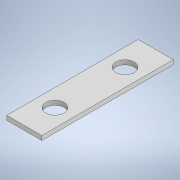
# Autodesk Inventor part: DrillSpacer
Saved by Autodesk Inventor 2022.1 (Build 261234020, 234B)
## iProperties
Created: 2023-10-25
Part Number: DrillSpacer
Material: Generic
Document SubType Name: Modeling
Designer: luke.macenski3281
Density: 1 g/cm^3
Appearance: Default
Author: luke.macenski3281
Autodesk Inventor part; units mm, degrees
ref_plane "YZ Plane" through (0, 0, 0) normal (1, 0, 0) x (0, 1, 0)
ref_plane "XZ Plane" through (0, 0, 0) normal (0, 1, 0) x (-1, 0, 0)
ref_plane "XY Plane" through (0, 0, 0) normal (0, 0, 1) x (1, 0, 0)
sketch "Sketch1" plane through (0, 0, 0) normal (0, 1, 0) x (-1, 0, 0)
  line L0 (0, 0) -> (10.16, 0)
  line L1 (10.16, 0) -> (10.16, -38.1)
  line L2 (10.16, -38.1) -> (0, -38.1)
  line L3 (0, -38.1) -> (0, 0)
  circle A0 centre (5.08, -8.89) radius 2.667
  circle A1 centre (5.08, -29.21) radius 2.667
  point P0 (5.08, -38.1)
  dimension "d0" = 10.16
  dimension "d1" = 38.1
  dimension "d2" = 5.334
  dimension "d3" = 5.334
  dimension "d4" = 5.08
  dimension "d5" = 5.08
  dimension "d6" = 20.32
  dimension "d7" = 8.89
  constraints: 8 end point, 2 centre point, 2 parallel, 1 horizontal, 1 midpoint, 1 perpendicular
  measures "d0" distance of L1.end L2.end
  measures "d1" distance between parallel lines of L0 L2
  measures "d2" diameter of A0
  measures "d3" diameter of A1
  measures "d4" horizontal distance of L0.start A0.centre
  measures "d5" horizontal distance of L0.start A1.centre
  measures "d6" distance of A1.centre A0.centre
  measures "d7" distance of point (5.08, -38.1) A1.centre
extrude "Extrusion1" add sketch "Sketch1" along normal blind 1.27
body "Solid1"
